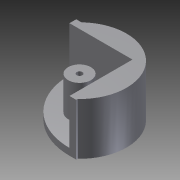
# Autodesk Inventor part: tv-mount
Saved by Autodesk Inventor 2012 (Build 160160000, 160)
## iProperties
Created: 2014-03-21
Part Number: tv-mount
Material: Default
Document SubType Name: Modeling
Designer: joe_000
Density: 1 g/cm^3
centerHoleDia: 2.500 mm
Author: joe_000
Autodesk Inventor part; units mm, degrees
ref_plane "YZ Plane" through (0, 0, 0) normal (1, 0, 0) x (0, 1, 0)
ref_plane "XZ Plane" through (0, 0, 0) normal (0, 1, 0) x (-1, 0, 0)
ref_plane "XY Plane" through (0, 0, 0) normal (0, 0, 1) x (1, 0, 0)
sketch "Sketch1" plane through (0, 0, 0) normal (0, 0, 1) x (1, 0, 0)
  arc A0 (-31, -3) -> (-3, -31) centre (-3, -3) ccw
  line L0 (-31, -3) -> (-31, 0)
  line L1 (-31, 0) -> (0, 0)
  line L2 (0, 0) -> (0, -31)
  line L3 (0, -31) -> (-3, -31)
  line L4 (-31, -3) -> (-3, -3)
  line L5 (-3, -3) -> (-3, -31)
  circle A1 centre (-14.34, -15.19) radius 5.05
  circle A2 centre (-14.34, -15.19) radius 1.25
  arc A3 (0, -30.38) -> (-28.68, 0) centre (-14.34, -15.19) ccw
  dimension "wallThickness" = 3
  dimension "d1" = 3
  dimension "width" = 31
  dimension "d3" = 31
  dimension "diameter" = 10.1
  dimension "d5" = 12.19
  dimension "d6" = 11.34
  dimension "centerHoleDia" = 2.5
  constraints: 12 end point, 5 point on circle, 4 centre point, 3 coincident, 3 parallel, 2 point on line, 1 perpendicular, 1 tangent, 1 vertical
  measures "wallThickness" distance of L0.start L0.end
  measures "d1" distance of L2.end L3.end
  measures "width" distance of L1.end L2.end
  measures "d3" distance of L0.end L1.end
  measures "diameter" diameter of A1
  measures "d5" distance from line of L4 A1.centre
  measures "d6" distance from line of L5 A1.centre
  measures "centerHoleDia" diameter of A2
extrude "Extrusion1" add sketch "Sketch1" against normal blind 3 contours L4 L5 A0 | L0 L1 L2 L3 L5 L4 | A3 L1 | L2 A3 | A1 | A2
extrude "Extrusion2" add sketch "Sketch1" along normal blind 20 contours L0 L1 L2 L3 L5 L4 | A3 L1 | L2 A3
extrude "Extrusion3" add sketch "Sketch1" along normal blind 15 contours A1 | A2
extrude "Extrusion7" cut sketch "Sketch1" along normal through all both and the other way through all contours A2
equation "\"d1\" = wallThickness"
equation "\"d3\" = width"
equation "\"d7\" = wallThickness"
body "Solid1"
